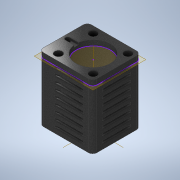
# Autodesk Inventor part: cylinder
Saved by Autodesk Inventor 2021.1 (Build 251245000, 245)
## iProperties
Created: 2020-08-30
Part Number: cylinder
Material: Aluminum 6061
Document SubType Name: Sheet Metal
Designer: Vamshi
Density: 2.7 g/cm^3
Sheet Metal Rule: Default
Appearance: Black Cast
Mass: 3204.09 g
Surface Area: 1935.26 cm^2
Volume: 1186.7 cm^3
Author: Vamshi
Autodesk Inventor part; units mm, degrees
ref_plane "YZ Plane" through (0, 0, 0) normal (1, 0, 0) x (0, 1, 0)
ref_plane "XZ Plane" through (0, 0, 0) normal (0, 1, 0) x (-1, 0, 0)
ref_plane "XY Plane" through (0, 0, 0) normal (0, 0, 1) x (1, 0, 0)
sketch "Sketch1" plane through (0, 0, 0) normal (0, 0, 1) x (1, 0, 0)
  line L0 (-60.96, 57.15) -> (45.72, 57.15)
  line L1 (55.88, 46.99) -> (55.88, -46.99)
  line L2 (45.72, -57.15) -> (-60.96, -57.15)
  line L3 (-71.12, -46.99) -> (-71.12, 46.99)
  line L4 (-99.4659, 0) -> (84.2259, 0) projected
  line L5 (0, -82.9559) -> (0, 82.9559) projected
  arc A0 (-60.96, 57.15) -> (-71.12, 46.99) centre (-60.96, 46.99) ccw
  arc A1 (55.88, 46.99) -> (45.72, 57.15) centre (45.72, 46.99) ccw
  arc A2 (45.72, -57.15) -> (55.88, -46.99) centre (45.72, -46.99) ccw
  arc A3 (-71.12, -46.99) -> (-60.96, -57.15) centre (-60.96, -46.99) ccw
  circle A4 centre (0, 0) radius 40.64
  point P0 (55.88, -57.15)
  point P1 (55.88, 57.15)
  point P2 (-71.12, -57.15)
  point P3 (-71.12, 0)
  dimension "d0" = 127
  dimension "d1" = 114.3
  dimension "d2" = 55.88
  dimension "d3" = 10.16
  dimension "d6" = 81.28
  constraints: 8 end point, 8 point on circle, 8 tangent, 7 point on line, 5 centre point, 3 equal radius, 2 parallel, 1 coincident, 1 horizontal, 1 midpoint, 1 perpendicular
  measures "d0" distance of point (55.88, -57.15) point (-71.12, -57.15)
  measures "d1" distance of point (55.88, 57.15) point (55.88, -57.15)
  measures "d2" distance between parallel lines of L5 L1
  measures "d3" radius of A0
  measures "d6" diameter of A4
extrude "Extrusion1" add sketch "Sketch1" along normal blind 157.48
extrude "Extrusion2" cut sketch "Sketch1" along normal blind 157.48 contours A4 L4 L5 | L5 L4 A4 | L5 A4 L4 | L4 A4 L5
sketch "Sketch2" plane through (0, 0, 157.48) normal (0, 0, 1) x (1, 0, 0)
  circle A0 centre (0, 0) radius 58.42 construction
  line L0 (0, 0) -> (45.72, 45.72) construction
  line L1 (0, 0) -> (64.6578, 0) construction
  circle A1 centre (41.3092, 41.3092) radius 8.89
  circle A2 centre (-41.3092, 41.3092) radius 8.89
  circle A3 centre (-41.3092, -41.3092) radius 8.89
  circle A4 centre (41.3092, -41.3092) radius 8.89
  dimension "d9" = 116.84
  dimension "d10" = 45
  dimension "d11" = 17.78
  dimension "d14" = 360
  constraints: 4 centre point, 4 end point, 1 coincident, 1 equal length, 1 horizontal, 1 point on line, 12 other
  measures "d10" angle of L1 L0
  measures "d11" diameter of A1
extrude "Extrusion3" cut sketch "Sketch2" against normal through all
sketch "Sketch3" plane through (0, 0, 157.48) normal (0, 0, 1) x (1, 0, 0)
  circle A0 centre (-60.96, 0) radius 5.08
  line L0 (-60.96, 5.08) -> (-31.75, 5.08)
  line L1 (-31.75, 5.08) -> (-31.75, -5.08)
  line L2 (-31.75, -5.08) -> (-60.96, -5.08)
  line L3 (-96.52, 0) -> (81.28, 0) projected
  point P0 (0, 0)
  point P1 (-31.75, 0)
  dimension "d18" = 10.16
  dimension "d19" = 60.96
  dimension "d20" = 10.16
  constraints: 6 end point, 2 point on circle, 1 centre point, 1 horizontal, 1 horizontal alignment, 1 midpoint, 1 parallel, 1 perpendicular, 1 point on line
  measures "d18" diameter of A0
  measures "d19" distance of point (0, 0) A0.centre
  measures "d20" distance of L0.end L1.end
extrude "Extrusion4" cut sketch "Sketch3" against normal through all contours L3 A0 | A0 L3
extrude "Extrusion5" cut sketch "Sketch3" against normal blind 5.08 contours L3 L1 L2 A0 | A0 L0 L1 L3
sketch "Sketch4" plane through (0, 0, 0) normal (0, 1, 0) x (-1, 0, 0)
  line L0 (45.72, 5.08) -> (-45.72, 5.08)
  line L1 (-45.72, 5.08) -> (-45.72, 0)
  line L2 (-45.72, 0) -> (45.72, 0)
  line L3 (45.72, 0) -> (45.72, 5.08)
  line L4 (0, -49.022) -> (0, 191.897) projected
  line L5 (-45.72, 0) -> (-55.88, 0) projected
  line L6 (60.96, 0) -> (-45.72, 0) projected
  line L7 (-45.72, 0) -> (-45.72, 157.48) projected
  line L8 (60.96, 157.48) -> (-45.72, 157.48) projected
  line L9 (60.96, 0) -> (60.96, 157.48) projected
  line L10 (40.64, 152.4) -> (55.88, 152.4) projected
  line L11 (55.88, 152.4) -> (55.88, 0) projected
  line L12 (55.88, 0) -> (40.64, 0) projected
  line L13 (40.64, 0) -> (40.64, 152.4) projected
  line L14 (71.12, 157.48) -> (71.12, 0) projected
  line L15 (71.12, 0) -> (66.04, 0) projected
  line L16 (66.04, 0) -> (66.04, 157.48) projected
  line L17 (66.04, 157.48) -> (71.12, 157.48) projected
  line L18 (-55.88, 0) -> (-55.88, 157.48) projected
  line L19 (-55.88, 157.48) -> (-40.64, 157.48) projected
  line L20 (-40.64, 157.48) -> (-40.64, 0) projected
  line L21 (-40.64, 0) -> (-55.88, 0) projected
  line L22 (45.72, 0) -> (96.52, 0)
  line L23 (96.52, 0) -> (96.52, 5.08)
  line L24 (96.52, 5.08) -> (45.72, 5.08)
  line L25 (45.72, 5.08) -> (45.72, 0)
  point P0 (0, 0)
  point P1 (0, 5.08)
  dimension "d25" = 91.44
  dimension "d26" = 5.08
  dimension "d27" = 50.8
  constraints: 16 end point, 4 parallel, 2 horizontal, 2 perpendicular, 2 point on line, 1 midpoint
  measures "d25" distance of L2.end L1.end
  measures "d26" distance of L1.end L0.end
  measures "d27" distance of L24.end L23.end
revolve "Revolution1" cut sketch "Sketch4" angle 360 about axis through (0, 0, -10) along (0, 0, 1) contours L24 L11 L6 L3 | L24 L9 L6 L11 | L24 L16 L22 L9 | L24 L14 L15 L16 | L24 L23 L22 L14
ref_plane "Work Plane1" through (0, 0, 144.78) normal (0, 0, 1) x (1, 0, 0)
sketch "Sketch5" plane through (0, 0, 144.78) normal (0, 0, 1) x (1, 0, 0)
  arc A0 (-60.96, 57.15) -> (-71.12, 46.99) centre (-60.96, 46.99) ccw
  line L0 (-60.96, 57.15) -> (45.72, 57.15)
  arc A1 (55.88, 46.99) -> (45.72, 57.15) centre (45.72, 46.99) ccw
  line L1 (55.88, 46.99) -> (55.88, -46.99)
  arc A2 (45.72, -57.15) -> (55.88, -46.99) centre (45.72, -46.99) ccw
  line L2 (45.72, -57.15) -> (-60.96, -57.15)
  arc A3 (-71.12, -46.99) -> (-60.96, -57.15) centre (-60.96, -46.99) ccw
  line L3 (-71.12, -46.99) -> (-71.12, 46.99)
  circle A4 centre (-60.96, 0) radius 5.08
  circle A5 centre (41.3092, -41.3092) radius 8.89
  circle A6 centre (-41.3092, -41.3092) radius 8.89
  circle A7 centre (41.3092, 41.3092) radius 8.89
  circle A8 centre (-41.3092, 41.3092) radius 8.89
  circle A9 centre (0, 0) radius 40.64
  constraints: 10 centre point, 8 end point, 8 point on circle
sketch "Sketch6" plane through (0, 0, 144.78) normal (0, 0, 1) x (1, 0, 0)
  arc A0 (55.88, 33.6969) -> (55.88, -33.6969) centre (106.68, 0) ccw
  line L0 (55.88, -46.99) -> (55.88, 46.99) projected
  arc A1 (-33.6969, 57.15) -> (33.6969, 57.15) centre (0, 107.95) ccw
  line L1 (45.72, 57.15) -> (-60.96, 57.15) projected
  arc A2 (33.6969, -57.15) -> (-33.6969, -57.15) centre (0, -107.95) ccw
  line L2 (-60.96, -57.15) -> (45.72, -57.15) projected
  line L3 (-40.3212, -5.08) -> (-60.96, -5.08) projected
  arc A3 (-60.96, 5.08) -> (-60.96, -5.08) centre (-60.96, 0) ccw projected
  line L4 (-60.96, 5.08) -> (-40.3212, 5.08) projected
  arc A4 (-40.3212, -5.08) -> (-40.3212, 5.08) centre (0, 0) ccw projected
  circle A5 centre (41.3092, -41.3092) radius 8.89 projected
  circle A6 centre (-41.3092, -41.3092) radius 8.89 projected
  circle A7 centre (41.3092, 41.3092) radius 8.89 projected
  circle A8 centre (-41.3092, 41.3092) radius 8.89 projected
  line L5 (55.88, -46.99) -> (55.88, 46.99) projected
  arc A9 (55.88, 46.99) -> (45.72, 57.15) centre (45.72, 46.99) ccw projected
  line L6 (45.72, 57.15) -> (-60.96, 57.15) projected
  arc A10 (-60.96, 57.15) -> (-71.12, 46.99) centre (-60.96, 46.99) ccw projected
  line L7 (-71.12, 46.99) -> (-71.12, -46.99) projected
  arc A11 (-71.12, -46.99) -> (-60.96, -57.15) centre (-60.96, -46.99) ccw projected
  line L8 (-60.96, -57.15) -> (45.72, -57.15) projected
  arc A12 (45.72, -57.15) -> (55.88, -46.99) centre (45.72, -46.99) ccw projected
  arc A13 (-60.96, 57.15) -> (-71.12, 46.99) centre (-60.96, 46.99) ccw projected
  line L9 (-60.96, 57.15) -> (45.72, 57.15) projected
  arc A14 (55.88, 46.99) -> (45.72, 57.15) centre (45.72, 46.99) ccw projected
  line L10 (55.88, 46.99) -> (55.88, -46.99) projected
  arc A15 (45.72, -57.15) -> (55.88, -46.99) centre (45.72, -46.99) ccw projected
  line L11 (45.72, -57.15) -> (-60.96, -57.15) projected
  arc A16 (-71.12, -46.99) -> (-60.96, -57.15) centre (-60.96, -46.99) ccw projected
  line L12 (-71.12, -46.99) -> (-71.12, 46.99) projected
  circle A17 centre (-60.96, 0) radius 5.08 projected
  circle A18 centre (41.3092, -41.3092) radius 8.89 projected
  circle A19 centre (-41.3092, -41.3092) radius 8.89 projected
  circle A20 centre (41.3092, 41.3092) radius 8.89 projected
  circle A21 centre (-41.3092, 41.3092) radius 8.89 projected
  circle A22 centre (0, 0) radius 40.64 projected
  dimension "d32" = 121.92
  dimension "d33" = 50.8
  dimension "d34" = 121.92
  dimension "d35" = 50.8
  dimension "d36" = 121.92
  dimension "d37" = 50.8
  constraints: 6 point on circle, 6 point on line, 3 centre point, 1 horizontal alignment, 1 vertical alignment
  measures "d32" diameter of A0
  measures "d33" distance from line of L0 A0.centre
  measures "d34" diameter of A1
  measures "d35" distance from line of L1 A1.centre
  measures "d36" diameter of A2
  measures "d37" distance from line of L2 A2.centre
extrude "Extrusion6" cut sketch "Sketch6" against normal blind 5.08 contours L0 A0 | A1 L1 | L2 A2
pattern_linear "Rectangular Pattern1" count 9 spacing 15.24 along (0, 0, -1) of "Extrusion6"
equation "\"BendRadius\" = Thickness"
equation "\"BendReliefWidth\" = Thickness"
equation "\"BendReliefDepth\" = 0.5 * Thickness"
equation "\"CornerReliefSize\" = 4 * Thickness"
equation "\"MinimumRemnant\" = 2 * Thickness"
equation "\"TransitionRadius\" = BendRadius"
equation "\"JacobiRadiusSize\" = BendRadius"
equation "\"GapSize\" = Thickness"
equation "\"Thickness\" = 3.048"
body "Solid1"
